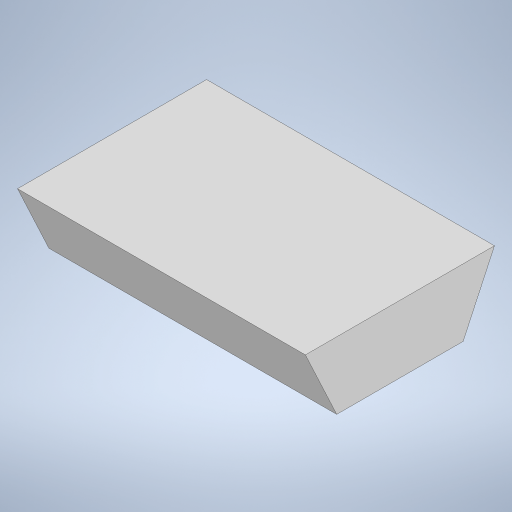
# Autodesk Inventor part: Bottom Sensor Mount
Saved by Autodesk Inventor 2023 (Build 270158000, 158)
## iProperties
Created: 2023-01-24
Part Number: Bottom Sensor Mount
Material: Generic
Document SubType Name: Modeling
Designer: Ahmed Nazir
Density: 1 g/cm^3
Appearance: Default
Author: Ahmed Nazir
Autodesk Inventor part; units mm, degrees
ref_plane "YZ Plane" through (0, 0, 0) normal (1, 0, 0) x (0, 1, 0)
ref_plane "XZ Plane" through (0, 0, 0) normal (0, 1, 0) x (-1, 0, 0)
ref_plane "XY Plane" through (0, 0, 0) normal (0, 0, 1) x (1, 0, 0)
sketch "Sketch1" plane through (0, 0, 0) normal (1, 0, 0) x (0, 1, 0)
  line L0 (0, 0) -> (0, -13.174)
  line L1 (0, -13.174) -> (7, -16.4382)
  line L2 (7, -16.4382) -> (7, 3.2642)
  line L3 (7, 3.2642) -> (0, 0)
  point P0 (0, -6.587)
  dimension "d0" = 13.174
  dimension "d1" = 65
  dimension "d2" = 65
  dimension "d8" = 7
  constraints: 8 end point, 1 midpoint, 1 parallel, 1 vertical
  measures "d0" distance of L0.start L0.end
  measures "d1" angle of L0 L3
  measures "d2" angle of L0 L1
  measures "d8" distance between parallel lines of L0 L2
extrude "Extrusion1" add sketch "Sketch1" along normal blind 30
body "Solid1"
